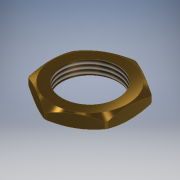
# Autodesk Inventor part: 4024-86
Saved by Autodesk Inventor 2019 (Build 230136000, 136)
## iProperties
Created: 2018-04-22
Part Number: 4024-86
Material: Brass
Document SubType Name: Modeling
Designer: IEUser
Density: 8.49 g/cm^3
Appearance: Brass - Polished
Author: IEUser
Autodesk Inventor part; units mm, degrees
ref_plane "YZ Plane" through (0, 0, 0) normal (1, 0, 0) x (0, 1, 0)
ref_plane "XZ Plane" through (0, 0, 0) normal (0, 1, 0) x (-1, 0, 0)
ref_plane "XY Plane" through (0, 0, 0) normal (0, 0, 1) x (1, 0, 0)
sketch "Body Cross Section" plane through (0, 0, 0) normal (0, 1, 0) x (-1, 0, 0)
  line L0 (-4.0415, -7) -> (-8.0829, 0)
  line L1 (-8.0829, 0) -> (-4.0415, 7)
  line L2 (-4.0415, 7) -> (4.0415, 7)
  line L3 (4.0415, 7) -> (8.0829, 0)
  line L4 (8.0829, 0) -> (4.0415, -7)
  line L5 (4.0415, -7) -> (-4.0415, -7)
  circle A0 centre (0, 0) radius 5
  dimension "d0" = 14
  dimension "d1" = 10
  constraints: 12 end point, 2 coincident, 1 centre point, 1 horizontal, 13 other
  measures "d0" distance between parallel lines of L2 L5
  measures "d1" diameter of A0
extrude "Body" add sketch "Body Cross Section" along normal blind 2.5
thread "Hole Thread" size "M10x0.75" class "6H" standard "ANSI Metric M Profile" full length
sketch "Body Chamfer Cross Section" plane through (0, 0, 0) normal (1, 0, 0) x (0, 1, 0)
  line L0 (3.5, -5) -> (3.5, -9)
  line L1 (3.5, -9) -> (-1, -9)
  line L2 (2.5, -7) -> (2.5, 0) projected
  line L3 (0, -7) -> (2.5, -7) projected
  line L4 (0, 0) -> (10, 0) construction
  line L5 (-1, -9) -> (-1, -5)
  line L6 (-1, -5) -> (1, -8.5)
  line L7 (1, -8.5) -> (1.5, -8.5)
  line L8 (1.5, -8.5) -> (3.5, -5)
  line L9 (0, 0) -> (0, -7) projected
  dimension "d7" = 1
  dimension "d8" = 4
  dimension "d9" = 2
  dimension "d11" = 10
  dimension "d14" = 0.5
  dimension "d15" = 1
  dimension "d16" = 0.5
  dimension "d17" = 4
  dimension "d18" = 1
  constraints: 14 end point, 2 horizontal, 2 parallel, 1 perpendicular
  measures "d7" distance between parallel lines of L2 L0
  measures "d8" distance of L0.start L0.end
  measures "d9" distance between parallel lines of L3 L1
  measures "d11" distance of L4.start L4.end
  measures "d14" distance between parallel lines of L1 L7
  measures "d15" distance between parallel lines of L9 L5
  measures "d16" distance of L6.end L7.end
  measures "d17" distance of L1.end L5.end
  measures "d18" distance from line of L2 L7.end
revolve "Body Chamfer" cut sketch "Body Chamfer Cross Section" angle 360 about axis through (0, 0, 0) along (0, 1, 0) contours L0 L1 L5 L6 L9 L3 L7 L8 L2 | L2 L3 L8 | L3 L9 L6
chamfer "Edge Chamfer" distance 0.25 angle 45 6 edges at (-8.0829, 1.25, 0) (-4.0415, 1.25, -7) (4.0415, 1.25, -7) (8.0829, 1.25, 0) (4.0415, 1.25, 7) (-4.0415, 1.25, 7)
equation "\"d17\" = d8"
body "Solid1"
